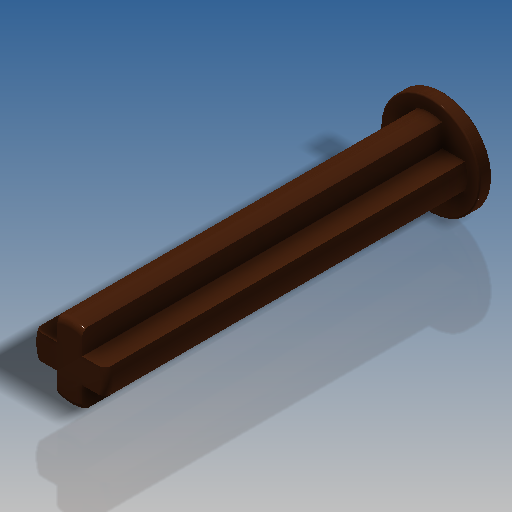
# Autodesk Inventor part: 24316-ReddishBrown
Saved by Autodesk Inventor 2019.4 (Build 234330000, 330)
## iProperties
Created: 2014-06-05
Part Number: 24316-ReddishBrown
Material: ABS Plastic
Document SubType Name: Modeling
Designer: D. Kohfeld
Density: 1.06 g/cm^3
Appearance: ReddishBrown
Mass: 0.334609 g
Surface Area: 5.00179 cm^2
Volume: 0.315669 cm^3
Author: D. Kohfeld
Autodesk Inventor part; units mm, degrees
ref_plane "YZ Plane" through (0, 0, 0) normal (1, 0, 0) x (0, 1, 0)
ref_plane "XZ Plane" through (0, 0, 0) normal (0, 1, 0) x (-1, 0, 0)
ref_plane "XY Plane" through (0, 0, 0) normal (0, 0, 1) x (1, 0, 0)
sketch "Sketch1" plane through (0, 0, 0) normal (0, 0, 1) x (1, 0, 0)
  circle A0 centre (0, 0) radius 2.4 construction
  line L0 (-0.8, 2.2627) -> (-0.8, 0.8)
  line L1 (-0.8, 0.8) -> (-2.2627, 0.8)
  line L2 (-2.2627, -0.8) -> (-0.8, -0.8)
  line L3 (-0.8, -0.8) -> (-0.8, -2.2627)
  line L4 (0.8, -2.2627) -> (0.8, -0.8)
  line L5 (0.8, -0.8) -> (2.2627, -0.8)
  line L6 (2.2627, 0.8) -> (0.8, 0.8)
  line L7 (0.8, 0.8) -> (0.8, 2.2627)
  arc A1 (0.8, 2.2627) -> (-0.8, 2.2627) centre (0, 0) ccw
  arc A2 (-2.2627, 0.8) -> (-2.2627, -0.8) centre (0, 0) ccw
  arc A3 (-0.8, -2.2627) -> (0.8, -2.2627) centre (0, 0) ccw
  arc A4 (2.2627, -0.8) -> (2.2627, 0.8) centre (0, 0) ccw
  dimension "d0" = 4.8
  dimension "d1" = 1.6
  constraints: 16 end point, 8 point on circle, 7 equal length, 4 centre point, 4 perpendicular, 3 parallel, 1 coincident, 1 vertical, 14 other
  measures "d1" distance between parallel lines of L0 L7
extrude "Extrusion1" add sketch "Sketch1" along normal mid plane 24
sketch "Sketch2" plane through (0, 0, -12) normal (0, 0, -1) x (-1, 0, 0)
  line L0 (0.8, 0.8) -> (0.8, 2.2627) projected
  arc A0 (0.8, 2.2627) -> (-0.8, 2.2627) centre (0, 0) ccw projected
  line L1 (-0.8, 2.2627) -> (-0.8, 0.8) projected
  line L2 (-0.8, 0.8) -> (-2.2627, 0.8) projected
  arc A1 (-2.2627, 0.8) -> (-2.2627, -0.8) centre (0, 0) ccw projected
  line L3 (-2.2627, -0.8) -> (-0.8, -0.8) projected
  line L4 (-0.8, -0.8) -> (-0.8, -2.2627) projected
  arc A2 (-0.8, -2.2627) -> (0.8, -2.2627) centre (0, 0) ccw projected
  line L5 (0.8, -2.2627) -> (0.8, -0.8) projected
  line L6 (0.8, -0.8) -> (2.2627, -0.8) projected
  arc A3 (2.2627, -0.8) -> (2.2627, 0.8) centre (0, 0) ccw projected
  line L7 (2.2627, 0.8) -> (0.8, 0.8) projected
  circle A4 centre (0, 0) radius 3.2
  dimension "d7" = 6.4
  constraints: 1 centre point, 1 coincident
  measures "d7" diameter of A4
extrude "Extrusion2" add sketch "Sketch2" against normal blind 0.8
fillet "Fillet1" radius 0.4 4 edges at (0, 2.4, 12) (-2.4, 0, 12) (0, -2.4, 12) (2.4, 0, 12)
fillet "Fillet1" radius 0.1 2 edges at (3.2, 0, -11.2) (3.2, 0, -12)
equation "\"d0\" = kd"
equation "\"d1\" = axlet"
equation "\"d2\" = 3 * lu"
equation "\"d7\" = tsd"
equation "\"d8\" = tsl"
equation "\"d4\" = tf"
equation "\"d10\" = lf"
equation "\"kd\" = 4.8"
equation "\"axlet\" = 1.6"
equation "\"lu\" = 8"
equation "\"tsd\" = 6.4"
equation "\"tsl\" = 0.8"
equation "\"tf\" = 0.4"
equation "\"lf\" = 0.1"
body "Solid1"
